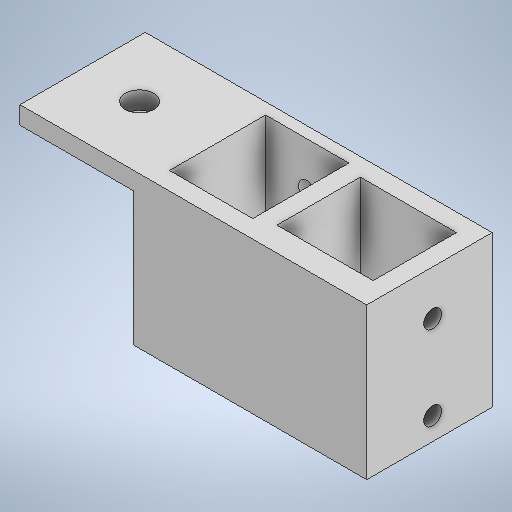
# Autodesk Inventor part: PluckMount
Saved by Autodesk Inventor 2025.1 (Build 291241000, 241)
## iProperties
Created: 2025-12-01
Part Number: PluckMount
Material: Generic
Document SubType Name: Modeling
Designer: Juxin
Density: 1 g/cm^3
Appearance: Default
Author: Juxin
Autodesk Inventor part; units mm, degrees
ref_plane "YZ Plane" through (0, 0, 0) normal (1, 0, 0) x (0, 1, 0)
ref_plane "XZ Plane" through (0, 0, 0) normal (0, 1, 0) x (-1, 0, 0)
ref_plane "XY Plane" through (0, 0, 0) normal (0, 0, 1) x (1, 0, 0)
sketch "Sketch1" plane through (0, 0, 0) normal (0, 1, 0) x (-1, 0, 0)
  line L0 (0, 0) -> (14.859, 0)
  line L1 (14.859, 0) -> (14.859, -17.145)
  line L2 (14.859, -17.145) -> (0, -17.145)
  line L3 (0, -17.145) -> (0, 0)
  line L4 (0, 0) -> (0, -1.143)
  line L5 (0, -1.143) -> (-3.175, -1.143)
  line L6 (-3.175, -1.143) -> (-20.32, -1.143)
  line L7 (-20.32, -1.143) -> (-20.32, -16.002)
  line L8 (-20.32, -16.002) -> (-3.175, -16.002)
  line L9 (-3.175, -16.002) -> (-3.175, -1.143)
  line L10 (14.859, 0) -> (14.859, 3.175)
  line L11 (14.859, 3.175) -> (18.034, 3.175)
  line L12 (-20.32, -1.143) -> (-23.495, -1.143)
  line L13 (-20.32, -16.002) -> (-20.32, -19.177)
  line L14 (-20.32, -19.177) -> (-23.495, -19.177)
  line L15 (18.034, 3.175) -> (-23.495, 3.175)
  line L16 (-23.495, 3.175) -> (-23.495, -19.177)
  line L17 (-23.495, -19.177) -> (18.034, -19.177)
  line L18 (18.034, -19.177) -> (18.034, 3.175)
  dimension "d0" = 14.859
  dimension "d1" = 17.145
  dimension "d2" = 1.143
  dimension "d3" = 3.175
  dimension "d4" = 17.145
  dimension "d5" = 14.859
  dimension "d6" = 3.175
  dimension "d7" = 3.175
  dimension "d8" = 3.175
  dimension "d34" = 3.175
  dimension "d35" = 3.175
  constraints: 38 end point, 6 parallel, 5 perpendicular, 4 horizontal, 2 point on line, 2 vertical
  measures "d0" distance of L1.end L2.end
  measures "d1" distance of L0.end L1.end
  measures "d2" distance of L0.start L4.end
  measures "d3" distance of L4.end L5.end
  measures "d4" distance of L8.end L7.end
  measures "d5" distance of L7.end L6.end
  measures "d6" distance of L0.end L10.end
  measures "d7" distance of L10.end L11.end
  measures "d8" distance of L6.end L12.end
  measures "d34" distance of L7.end L13.end
  measures "d35" distance of L13.end L14.end
extrude "Extrusion1" add sketch "Sketch1" along normal blind 25.4 contours L3 L5 L6 L12 L16 L15 L10 L0 | L10 L11 L18 L17 L13 L8 L9 L5 L3 L2 L1 | L7 L13 L14 L16 L12
sketch "Sketch2" plane through (23.495, 0, 1.5875) normal (1, 0, 0) x (0, 0, -1)
  line L0 (17.5895, 25.4) -> (2.7305, 25.4) projected
  line L1 (10.16, 25.4) -> (10.16, 17.399)
  circle A0 centre (10.16, 17.399) radius 1.5875
  line L2 (10.16, 17.399) -> (10.16, 2.413)
  circle A1 centre (10.16, 2.413) radius 1.5875
  point P0 (1.5875, 0)
  dimension "d13" = 8.001
  dimension "d14" = 3.175
  dimension "d15" = 14.986
  dimension "d16" = 3.175
  constraints: 4 end point, 2 centre point, 2 coincident, 2 vertical, 1 midpoint
  measures "d13" distance of L1.start L1.end
  measures "d14" diameter of A0
  measures "d15" distance of L2.start L2.end
  measures "d16" diameter of A1
extrude "Extrusion2" cut sketch "Sketch2" against normal blind 9.525
sketch "Sketch3" plane through (19.05, 0, -19.177) normal (0, 0, -1) x (-1, 0, 0)
  line L0 (33.909, 0) -> (33.909, 25.4) projected
  line L1 (19.05, 0) -> (19.05, 25.4) projected
  line L2 (33.909, 25.4) -> (19.05, 25.4)
  line L3 (26.4795, 25.4) -> (26.4795, 17.399)
  circle A0 centre (26.4795, 17.399) radius 1.5875
  line L4 (26.4795, 17.399) -> (26.4795, 2.413)
  circle A1 centre (26.4795, 2.413) radius 1.5875
  dimension "d19" = 8.001
  dimension "d20" = 3.175
  dimension "d21" = 14.986
  dimension "d22" = 3.175
  constraints: 6 end point, 2 centre point, 2 coincident, 2 vertical, 1 midpoint, 1 perpendicular
  measures "d19" distance of L3.start L3.end
  measures "d20" diameter of A0
  measures "d21" distance of L4.start L4.end
  measures "d22" diameter of A1
extrude "Extrusion3" cut sketch "Sketch3" against normal blind 9.525
move faces "Move1" translate (0, -1.5875, 0) faces at (1.8203, 0, 2.1167)
sketch "Sketch4" plane through (-18.034, 25.4, -17.4625) normal (-1, 0, 0) x (0, 0, 1)
  line L0 (19.05, 0) -> (0, 0)
  line L1 (20.6375, -26.9875) -> (20.6375, 0) projected
  line L2 (-1.7145, -26.9875) -> (-1.7145, 0) projected
  line L3 (20.6375, 0) -> (-1.7145, 0)
  line L4 (-1.7145, 0) -> (-1.7145, -3.175)
  line L5 (-1.7145, -3.175) -> (20.6375, -3.175)
  line L6 (20.6375, -3.175) -> (20.6375, 0)
  point P0 (17.4625, -25.4)
  point P1 (20.6375, -3.175)
  dimension "d36" = 3.175
  constraints: 10 end point, 2 horizontal, 2 parallel, 1 perpendicular, 1 point on line
  measures "d36" distance of L4.end L3.end
extrude "Extrusion4" add sketch "Sketch4" along normal blind 20.32
sketch "Sketch5" plane through (-15.1765, 25.4, -17.4625) normal (0, -1, 0) x (1, 0, 0)
  line L0 (-23.1775, 20.6375) -> (-23.1775, -1.7145) projected
  line L1 (0.3175, 17.4625) -> (0.3175, 0.3175) projected
  line L2 (-23.1775, 9.4615) -> (0.3175, 9.4615) construction
  line L3 (-23.1775, 9.4615) -> (-2.8575, 9.4615)
  line L4 (-2.8575, -1.7145) -> (-2.8575, 20.6375) projected
  circle A0 centre (-13.0175, 9.4615) radius 2.54
  point P0 (15.1765, 17.4625)
  dimension "d39" = 5.08
  constraints: 4 end point, 3 midpoint, 1 centre point, 1 horizontal
  measures "d39" diameter of A0
extrude "Extrusion5" cut sketch "Sketch5" along normal blind 14.605
body "Solid1"
